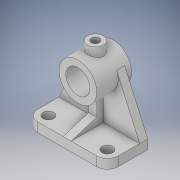
# Autodesk Inventor part: 練習一
Saved by Autodesk Inventor 2017 (Build 210142000, 142)
## iProperties
Part Number: 練習一
Material: 一般
Document SubType Name: Modeling
Designer: user
Density: 1 g/cm^3
Appearance: 預設
Author: user
Autodesk Inventor part; units mm, degrees
ref_plane "YZ Plane" through (0, 0, 0) normal (1, 0, 0) x (0, 1, 0)
ref_plane "XZ Plane" through (0, 0, 0) normal (0, 1, 0) x (-1, 0, 0)
ref_plane "XY Plane" through (0, 0, 0) normal (0, 0, 1) x (1, 0, 0)
sketch "草圖1" plane through (0, 0, 0) normal (0, 1, 0) x (-1, 0, 0)
  line L0 (30, -15) -> (-30, -15)
  line L1 (-30, -15) -> (-30, 15)
  line L2 (-30, 15) -> (30, 15)
  line L3 (30, 15) -> (30, -15)
  line L4 (30, -15) -> (-30, 15) construction
  line L5 (-30, -15) -> (30, 15) construction
  point P0 (0, 0)
  dimension "d0" = 60
  dimension "d1" = 30
  constraints: 12 end point, 2 midpoint, 2 parallel, 1 horizontal, 1 perpendicular
  measures "d0" distance of L0.start L0.end
  measures "d1" distance of L0.end L1.end
extrude "擠出1" add sketch "草圖1" along normal blind 7
fillet "圓角1" radius 8 2 edges at (30, 3.5, 15) (-30, 3.5, 15)
ref_plane "工作平面3" through (30, 0, -19) normal (0, 0, -1) x (-1, 0, 0)
sketch "草圖4" plane through (30, 0, -19) normal (0, 0, -1) x (-1, 0, 0)
  line L0 (30, 0) -> (30, 40) construction
  line L1 (60, 0) -> (0, 0) projected
  circle A0 centre (30, 40) radius 9
  circle A1 centre (30, 40) radius 14
  dimension "d15" = 40
  dimension "d16" = 18
  dimension "d17" = 28
  constraints: 2 centre point, 2 coincident, 2 end point, 1 vertical
  measures "d15" distance from line of L0.end L1
  measures "d16" diameter of A0
  measures "d17" diameter of A1
extrude "擠出3" add sketch "草圖4" against normal blind 26
sketch "草圖5" plane through (30, 0, -15) normal (0, 0, -1) x (-1, 0, 0)
  circle A0 centre (30, 40) radius 14 projected
  line L0 (0, 7) -> (17.2082, 45.6895)
  line L1 (30, 40) -> (30, 22.7943)
  line L2 (60, 7) -> (42.7918, 45.6895)
  line L3 (0, 0) -> (0, 7) projected
  line L4 (60, 7) -> (0, 7)
  arc A1 (17.2082, 45.6895) -> (42.7918, 45.6895) centre (30, 40) ccw
  point P0 (30, 0)
  constraints: 10 end point, 2 point on circle, 1 centre point, 1 coincident, 1 perpendicular, 1 symmetric about line, 1 vertical, 4 other
extrude "擠出4" add sketch "草圖5" against normal blind 6 contours A0 L2 L4 L0
ref_plane "工作平面4" through (0, 60, 0) normal (0, 1, 0) x (1, 0, 0)
sketch "草圖6" plane through (0, 60, 0) normal (0, 1, 0) x (1, 0, 0)
  circle A0 centre (0, 6) radius 6
  line L0 (-14, 19) -> (14, 19) projected
  line L1 (0, 0) -> (0, 6.6059)
  dimension "d24" = 12
  dimension "d25" = 13
  constraints: 2 end point, 2 vertical, 1 point on line, 1 vertical alignment, 2 other
  measures "d25" distance from line of L0 point (0, 6)
extrude "擠出5" add sketch "草圖6" against normal up to next
sketch "草圖7" plane through (0, 60, -6) normal (0, 1, 0) x (1, 0, 0)
  circle A0 centre (0, 0) radius 6 projected
  circle A1 centre (0, 0) radius 3
  point P0 (0, -6)
  dimension "d28" = 6
  constraints: 1 centre point, 1 coincident, 1 vertical alignment
  measures "d28" diameter of A1
extrude "擠出6" cut sketch "草圖7" against normal up to next contours A1
sketch "草圖8" plane through (0, 7, 0) normal (0, 1, 0) x (1, 0, 0)
  arc A0 (-30, -7) -> (-22, -15) centre (-22, -7) ccw projected
  circle A1 centre (-22, -7) radius 4
  arc A2 (22, -15) -> (30, -7) centre (22, -7) ccw projected
  circle A3 centre (22, -7) radius 4
  point P0 (0, 0)
  dimension "d31" = 8
  dimension "d32" = 8
  constraints: 2 centre point, 2 coincident
  measures "d31" diameter of A1
  measures "d32" diameter of A3
extrude "擠出7" cut sketch "草圖8" against normal up to next
sketch "草圖9" plane through (0, 0, 0) normal (1, 0, 0) x (0, 1, 0)
  line L0 (7, 15) -> (7, 7) projected
  line L1 (7, 15) -> (13, -4)
  line L2 (13, -4) -> (26, -4)
  line L3 (26, -19) -> (26, 7) projected
  line L4 (7, -9) -> (45.6895, -9) projected
  point P0 (0, 0)
  dimension "d35" = 6
  dimension "d36" = 5
  constraints: 4 end point, 1 horizontal, 1 point on line
  measures "d35" distance from line of L1.end L0
  measures "d36" distance between parallel lines of L4 L2
extrude "肋1" add sketch "草圖9" along normal mid plane 6 rib yes fills toward (7.05, 11) open curves L0 L1 L2
